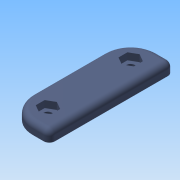
# Autodesk Inventor part: накладка на петлю
Saved by Autodesk Inventor 2017 (Build 210142000, 142)
## iProperties
Part Number: накладка на петлю
Material: Типовые
Document SubType Name: Modeling
Designer: Max
Mass: 2.37821 g
Surface Area: 17.5843 cm^2
Volume: 2.37821 cm^3
Density: 1 g/cm^3
Appearance: Резина — синяя
Author: Max
Autodesk Inventor part; units mm, degrees
ref_plane "YZ Plane" through (0, 0, 0) normal (1, 0, 0) x (0, 1, 0)
ref_plane "XZ Plane" through (0, 0, 0) normal (0, 1, 0) x (-1, 0, 0)
ref_plane "XY Plane" through (0, 0, 0) normal (0, 0, 1) x (1, 0, 0)
sketch "Эскиз1" plane through (0, 0, 0) normal (0, 0, 1) x (1, 0, 0)
  line L0 (123.2502, 86.3215) -> (123.2502, 112.3215) projected
  circle A0 centre (130.7502, 114.3215) radius 1.5 projected
  circle A1 centre (130.7502, 84.3215) radius 1.5 projected
  line L1 (132.7502, 121.8215) -> (144.7502, 121.8215) projected
  arc A2 (132.7502, 121.8215) -> (123.2502, 112.3215) centre (132.7502, 112.3215) ccw projected
  arc A3 (123.2502, 86.3215) -> (132.7502, 76.8215) centre (132.7502, 86.3215) ccw projected
  line L2 (138.7502, 76.8215) -> (132.7502, 76.8215) projected
  line L3 (138.7502, 88.4715) -> (138.7502, 76.8215) projected
  line L4 (138.7502, 111.4715) -> (138.7502, 98.6715) projected
  line L5 (144.5002, -126.5097) -> (144.5002, 144.1144) projected
  line L6 (138.7502, 76.8215) -> (138.7502, 121.8215)
  point P0 (0, 0)
  constraints: 2 end point, 1 midpoint
extrude "Выдавливание1" add sketch "Эскиз1" along normal blind 4
fillet "Сопряжение1" radius 2 6 edges at (123.2502, 99.3215, 4) (126.0327, 79.604, 4) (135.7502, 76.8215, 4) (135.7502, 121.8215, 4) (126.0327, 119.039, 4) (138.7502, 99.3215, 4)
fillet "Сопряжение2" radius 2 4 edges at (138.7502, 121.8215, 1) (138.1644, 121.2357, 3.4142) (138.7502, 76.8215, 1) (138.1644, 77.4073, 3.4142)
sketch "Эскиз2" plane through (0, 0, 4) normal (0, 0, 1) x (1, 0, 0)
  circle A0 centre (130.7502, 114.3215) radius 1.5 projected
  line L0 (130.7502, 117.5547) -> (133.5502, 115.9381)
  line L1 (133.5502, 115.9381) -> (133.5502, 112.7049)
  line L2 (133.5502, 112.7049) -> (130.7502, 111.0883)
  line L3 (130.7502, 111.0883) -> (127.9502, 112.7049)
  line L4 (127.9502, 112.7049) -> (127.9502, 115.9381)
  line L5 (127.9502, 115.9381) -> (130.7502, 117.5547)
  circle A1 centre (130.7502, 84.3215) radius 1.5 projected
  line L6 (130.7502, 87.5547) -> (133.5502, 85.9381)
  line L7 (133.5502, 85.9381) -> (133.5502, 82.7049)
  line L8 (133.5502, 82.7049) -> (130.7502, 81.0883)
  line L9 (130.7502, 81.0883) -> (127.9502, 82.7049)
  line L10 (127.9502, 82.7049) -> (127.9502, 85.9381)
  line L11 (127.9502, 85.9381) -> (130.7502, 87.5547)
  point P0 (0, 0)
  dimension "d4" = 3
  dimension "d5" = 5.6
  dimension "d6" = 5.6
  constraints: 24 end point, 2 coincident, 26 other
  measures "d4" diameter of A0
  measures "d5" distance between parallel lines of L1 L4
  measures "d6" distance between parallel lines of L7 L10
extrude "Выдавливание2" cut sketch "Эскиз2" against normal blind 2.5
